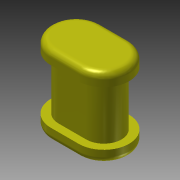
# Autodesk Inventor part: Antivibrador raqueta
Saved by Autodesk Inventor 2014 (Build 180170000, 170)
## iProperties
Created: 2015-03-22
Part Number: Antivibrador raqueta
Material: Generic
Document SubType Name: Modeling
Designer: Rubén
Density: 1 g/cm^3
Appearance: Yellow
Author: Rubén
Autodesk Inventor part; units mm, degrees
ref_plane "YZ Plane" through (0, 0, 0) normal (1, 0, 0) x (0, 1, 0)
ref_plane "XZ Plane" through (0, 0, 0) normal (0, 1, 0) x (-1, 0, 0)
ref_plane "XY Plane" through (0, 0, 0) normal (0, 0, 1) x (1, 0, 0)
sketch "Sketch1" plane through (0, 0, 0) normal (0, 1, 0) x (-1, 0, 0)
  line L0 (0, 0) -> (12.4, 0)
  line L1 (12.4, 0) -> (12.4, 8)
  line L2 (12.4, 8) -> (0, 8)
  line L3 (0, 8) -> (0, 0)
  dimension "d0" = 12.4
  dimension "d1" = 8
  constraints: 8 end point, 2 parallel, 1 horizontal, 1 perpendicular
  measures "d0" distance of L0.start L0.end
  measures "d1" distance of L0.end L1.end
extrude "Extrusion1" add sketch "Sketch1" along normal blind 6.3
fillet "Fillet1" radius 4 4 edges at (0, 3.15, 8) (0, 3.15, 0) (-12.4, 3.15, 8) (-12.4, 3.15, 0)
sketch "Sketch2" plane through (0, 6.3, 0) normal (0, 1, 0) x (1, 0, 0)
  arc A0 (-8.4, 0) -> (-8.4, -8) centre (-8.4, -4) ccw projected
  line L0 (-8.4, -8) -> (-4, -8) projected
  arc A1 (-4, -8) -> (-4, 0) centre (-4, -4) ccw projected
  line L1 (-4, 0) -> (-8.4, 0) projected
  arc A2 (-8.4, -1.2) -> (-8.4, -6.8) centre (-8.4, -4) ccw
  line L2 (-8.4, -6.8) -> (-4, -6.8)
  arc A3 (-4, -6.8) -> (-4, -1.2) centre (-4, -4) ccw
  line L3 (-4, -1.2) -> (-8.4, -1.2)
  point P0 (0, 0)
  dimension "d5" = 1.2
  constraints: 4 end point, 4 point on circle, 2 centre point, 3 other
  measures "d5" distance between parallel lines of L3 L1
extrude "Extrusion2" cut sketch "Sketch2" against normal blind 4.3
fillet "Fillet2" radius 1 8 edges at (-6.2, 0, 0) (-11.2285, 0, 6.8285) (-11.2285, 0, 1.1715) (-12.4, 0, 4) (-6.2, 0, 8) (-1.1715, 0, 1.1715) (0, 0, 4) (-1.1715, 0, 6.8285)
mirror "Mirror1" about plane through (-6.2, 6.3, 4) normal (0, 1, 0)
body "Solid1"
